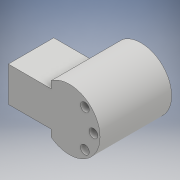
# Autodesk Inventor part: enganche_servo
Saved by Autodesk Inventor 2018 (Build 220112000, 112)
## iProperties
Created: 2018-04-15
Part Number: enganche_servo
Material: Genérico
Document SubType Name: Modeling
Designer: se_ma
Density: 1 g/cm^3
Appearance: Valor por defecto
Author: se_ma
Autodesk Inventor part; units mm, degrees
ref_plane "YZ Plane" through (0, 0, 0) normal (1, 0, 0) x (0, 1, 0)
ref_plane "XZ Plane" through (0, 0, 0) normal (0, 1, 0) x (-1, 0, 0)
ref_plane "XY Plane" through (0, 0, 0) normal (0, 0, 1) x (1, 0, 0)
sketch "Boceto1" plane through (0, 0, 0) normal (0, 1, 0) x (-1, 0, 0)
  line L0 (8.5, 0) -> (21, 0) construction
  line L1 (21, -7) -> (2.0913, -7)
  line L2 (21, -7) -> (27, -7)
  line L3 (21, 7) -> (27, 7)
  line L4 (27, 7) -> (27, -7)
  line L5 (27, -7) -> (32, -7)
  line L6 (32, -7) -> (32, 7)
  line L7 (32, 7) -> (27, 7)
  circle A0 centre (29.5, 0) radius 1
  line L8 (2.0913, -7) -> (2.0913, 7)
  line L9 (2.0913, -7) -> (16.0913, -7) construction
  line L10 (2.0913, 7) -> (21.0913, 7)
  line L11 (2.0913, -7) -> (-2.9087, -7)
  line L12 (2.0913, -7) -> (7.0913, -7) construction
  line L13 (-2.9087, -7) -> (-2.9087, 7)
  line L14 (-2.9087, 7) -> (2.0913, 7)
  circle A1 centre (-0.4087, 0) radius 1
  line L15 (2.0913, -7) -> (2.0913, 7)
  point P0 (0, 0)
  point P1 (0, 0)
  point P2 (0, 0)
  point P3 (0, 0)
  dimension "d3" = 6
  dimension "d5" = 5
  dimension "d6" = 14
  dimension "d7" = 2
  dimension "d8" = 14
  dimension "d9" = 90
  dimension "d10" = 19
  dimension "d11" = 5
  dimension "d12" = 180
  dimension "d13" = 14
  dimension "d14" = 2
  constraints: 32 end point, 5 horizontal, 3 perpendicular, 2 centre point, 2 equal length, 2 point on line, 1 collinear
  measures "d3" distance of L1.start L4.end
  measures "d5" distance of L4.end L5.end
  measures "d6" distance of L5.end L6.end
  measures "d7" diameter of A0
  measures "d8" distance of L11.start L14.end
  measures "d9" angle of L9 L8
  measures "d10" distance of L14.end L10.end
  measures "d11" distance of L11.start L11.end
  measures "d12" angle of L11 L12
  measures "d13" distance of L11.end L14.start
  measures "d14" diameter of A1
extrude "Extrusión1" add sketch "Boceto1" along normal blind 18 contours L11 L13 L14 L8 | L4 L7 L6 L5
sketch "Boceto2" plane through (0, 0, 0) normal (0, -1, 0) x (1, 0, 0)
  line L0 (2.9087, 10) -> (-32, 10)
  line L1 (-32, 10) -> (-35, 10)
  line L2 (-35, 10) -> (-35, -7)
  line L3 (-35, -7) -> (-35, -10)
  line L4 (-35, -10) -> (2.9087, -10)
  line L5 (2.9087, -10) -> (5.9087, -10)
  line L6 (5.9087, -10) -> (5.9087, 10)
  line L7 (5.9087, 10) -> (2.9087, 10)
  line L8 (-2.0913, -7) -> (-27, -7)
  line L9 (-27, 7) -> (-2.0913, 7)
  line L10 (-2.0913, 7) -> (2.9087, 7)
  line L11 (2.9087, 7) -> (2.9087, -7) projected
  line L12 (2.9087, 7) -> (2.9087, -7)
  line L13 (2.9087, -7) -> (-2.0913, -7) projected
  line L14 (2.9087, -7) -> (-2.0913, -7)
  line L15 (-32, 7) -> (-27, 7) projected
  line L16 (-27, 7) -> (-32, 7)
  line L17 (-32, -7) -> (-32, 7) projected
  line L18 (-32, 7) -> (-32, -7)
  line L19 (-27, -7) -> (-32, -7) projected
  line L20 (-32, -7) -> (-27, -7)
  point P0 (0, 0)
  dimension "d21" = 3
  dimension "d22" = 3
  dimension "d23" = 3
  constraints: 32 end point, 7 perpendicular, 3 point on line, 2 collinear, 1 horizontal
  measures "d21" distance of L0.end L1.end
  measures "d22" distance of L2.end L3.end
  measures "d23" distance of L4.end L5.end
extrude "Extrusión2" add sketch "Boceto2" against normal blind 23
sketch "Boceto3" plane through (0, 0, 0) normal (0, -1, 0) x (1, 0, 0)
  line L0 (5.9087, 10) -> (-35, 10) projected
  line L1 (5.9087, 10) -> (-35, 10)
  line L2 (-35, 10) -> (-35, -10) projected
  line L3 (-35, 10) -> (-35, -10)
  line L4 (-35, -10) -> (5.9087, -10)
  line L5 (5.9087, -10) -> (5.9087, 10) projected
  line L6 (5.9087, -10) -> (5.9087, 10)
  point P0 (0, 0)
  constraints: 8 end point, 2 collinear, 2 perpendicular
extrude "Extrusión3" add sketch "Boceto3" along normal blind 3
sketch "Boceto4" plane through (0, 23, 0) normal (0, 1, 0) x (1, 0, 0)
  circle A0 centre (0.4087, 0) radius 1 projected
  point P0 (0, 0)
extrude "Extrusión4" add sketch "Boceto4" along normal blind 15
sketch "Boceto5" plane through (0.4087, 38, 0) normal (0, 1, 0) x (1, 0, 0)
  circle A0 centre (-0.4087, 0) radius 10
  circle A1 centre (-0.4087, 0) radius 17.5
  line L0 (-35.4087, 10) -> (5.5, 10) projected
  line L1 (-35.4087, 10) -> (-35.4087, -10) projected
  line L2 (-35.4087, 10) -> (-35.4087, 14)
  line L3 (-35.4087, 14) -> (-10.9087, 14)
  line L4 (-10.9087, 14) -> (-5.5098, 8.6011)
  line L5 (-10.9087, 14) -> (-3.2735, 14) construction
  line L6 (5.5, -10) -> (-35.4087, -10) projected
  line L7 (-35.4087, -10) -> (-35.4087, -14)
  line L8 (-35.4087, -14) -> (-10.9087, -14)
  line L9 (-10.9087, -14) -> (-5.5098, -8.6011)
  line L10 (-10.9087, -14) -> (-3.2735, -14) construction
  dimension "d32" = 20
  dimension "d33" = 35
  dimension "d35" = 4
  dimension "d36" = 45
  dimension "d37" = 4
  dimension "d38" = 45
  constraints: 16 end point, 4 point on circle, 2 centre point, 2 coincident, 2 equal length, 2 horizontal, 2 perpendicular, 2 vertical
  measures "d32" diameter of A0
  measures "d33" diameter of A1
  measures "d35" distance of L0.start L2.end
  measures "d36" angle of L4 L5
  measures "d37" distance of L1.end L7.end
  measures "d38" angle of L10 L9
extrude "Extrusión5" add sketch "Boceto5" against normal blind 15 contours L4 L0 A0 | A0 L6 L9 | L0 L4 A1 L9 L6 A0 picked at (-3.4554, 12.4332)
sketch "Boceto6" plane through (0.4087, 38, 0) normal (0, 1, 0) x (1, 0, 0)
  circle A0 centre (0, 0) radius 1 projected
  circle A1 centre (0, 0) radius 1
  point P0 (-0.4087, 0)
  constraints: 1 centre point, 1 coincident
extrude "Extrusión6" cut sketch "Boceto6" against normal blind 15
sketch "Boceto7" plane through (0.4087, 23, 0) normal (0, -1, 0) x (1, 0, 0)
  circle A0 centre (-0.4087, 0) radius 17.5
  circle A1 centre (-0.4087, 0) radius 10
  line L0 (5.5, 8.0677) -> (5.5, -8.0677) projected
  arc A2 (-0.4087, -10) -> (5.5, -8.0677) centre (-0.4087, 0) ccw projected
  line L1 (5.5, 8.0677) -> (5.5, 10)
  line L2 (-35.4087, 10) -> (-6.9087, 10) projected
  line L3 (5.5, 10) -> (-6.9087, 10)
  line L4 (5.5, -8.0677) -> (5.5, -10) projected
  line L5 (5.5, -8.0677) -> (5.5, -10)
  line L6 (-0.4087, -10) -> (-6.9087, -10) projected
  line L7 (5.5, -10) -> (-6.9087, -10)
  arc A3 (-10.9087, -14) -> (-10.9087, 14) centre (-0.4087, 0) ccw projected
  line L8 (-10.9087, 14) -> (-10.9087, 10)
  line L9 (5.5, 10) -> (-35.4087, 10) projected
  line L10 (-10.9087, -14) -> (-10.9087, -10)
  line L11 (-10.9087, -10) -> (-6.9087, -10)
  line L12 (-6.9087, -10) -> (-35.4087, -10) projected
  dimension "d43" = 20
  constraints: 14 end point, 3 collinear, 2 coincident, 2 point on line, 2 vertical, 1 centre point, 1 point on circle, 2 other
  measures "d43" diameter of A1
extrude "Extrusión7" add sketch "Boceto7" along normal blind 26 contours A0 L10 L11 L6 L7 L4 A1 L1 L3 L2 L8 | A1 L0 picked at (8.0064, 0)
sketch "Boceto8" plane through (0.4087, 38, 0) normal (0, 1, 0) x (1, 0, 0)
  line L0 (-0.4087, 0) -> (13.3413, 0)
  line L1 (-0.4087, 0) -> (8.4296, -10.5331)
  line L2 (-0.4087, 0) -> (13.3413, 0) construction
  line L3 (-0.4087, 0) -> (8.4296, 10.5331)
  line L4 (-0.4087, 0) -> (13.3413, 0) construction
  circle A0 centre (13.3413, 0) radius 1.75
  circle A1 centre (8.4296, -10.5331) radius 1.75
  circle A2 centre (8.4296, 10.5331) radius 1.75
  dimension "d46" = 13.75
  dimension "d47" = 13.75
  dimension "d48" = 50
  dimension "d49" = 13.75
  dimension "d50" = 50
  dimension "d51" = 3.5
  dimension "d52" = 3.5
  dimension "d53" = 3.5
  constraints: 10 end point, 3 centre point, 3 horizontal, 2 coincident, 2 equal length, 1 point on line
  measures "d46" distance of L0.start L0.end
  measures "d47" distance of L0.start L1.end
  measures "d48" angle of L1 L2
  measures "d49" distance of L0.start L3.end
  measures "d50" angle of L4 L3
  measures "d51" diameter of A0
  measures "d52" diameter of A1
  measures "d53" diameter of A2
extrude "Extrusión8" cut sketch "Boceto8" against normal blind 41
sketch "Boceto9" plane through (0, -3, 0) normal (0, -1, 0) x (1, 0, 0)
  circle A0 centre (8.8383, 10.5331) radius 1.75 projected
  circle A1 centre (8.8383, 10.5331) radius 2.5
  circle A2 centre (13.75, 0) radius 1.75 projected
  circle A3 centre (13.75, 0) radius 2.5
  circle A4 centre (8.8383, -10.5331) radius 1.75 projected
  circle A5 centre (8.8383, -10.5331) radius 2.5
  point P0 (0, 0)
  dimension "d56" = 5
  dimension "d57" = 5
  dimension "d58" = 5
  constraints: 3 centre point, 3 coincident
  measures "d56" diameter of A1
  measures "d57" diameter of A3
  measures "d58" diameter of A5
extrude "Extrusión9" cut sketch "Boceto9" against normal blind 36
